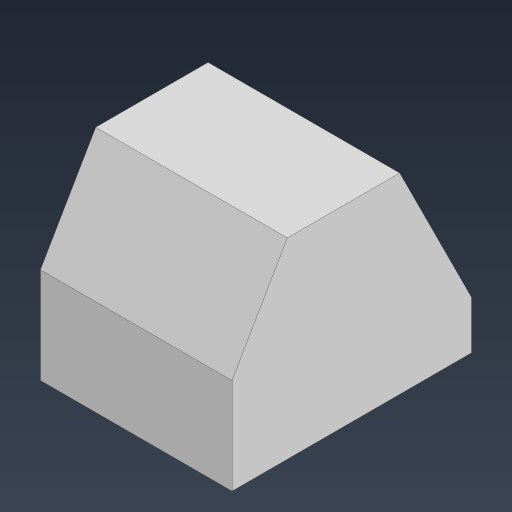
# Autodesk Inventor part: 3D Model
Saved by Autodesk Inventor 2024 (Build 280153000, 153)
## iProperties
Created: 2024-03-05
Part Number: 3D Model
Material: Genérico
Document SubType Name: Modeling
Designer: Administrator
Density: 1 g/cm^3
Appearance: Padrão
Author: Administrator
Autodesk Inventor part; units mm, degrees
ref_plane "YZ Plane" through (0, 0, 0) normal (1, 0, 0) x (0, 1, 0)
ref_plane "XZ Plane" through (0, 0, 0) normal (0, 1, 0) x (-1, 0, 0)
ref_plane "XY Plane" through (0, 0, 0) normal (0, 0, 1) x (1, 0, 0)
sketch "Esboço1" plane through (0, 0, 0) normal (0, 1, 0) x (-1, 0, 0)
  line L0 (20, -25) -> (-20, -25)
  line L1 (-20, -25) -> (-20, 25)
  line L2 (-20, 25) -> (20, 25)
  line L3 (20, 25) -> (20, -25)
  line L4 (20, -25) -> (-20, 25) construction
  line L5 (-20, -25) -> (20, 25) construction
  point P0 (0, 0)
  dimension "d0" = 40
  dimension "d1" = 50
  constraints: 12 end point, 2 midpoint, 2 parallel, 1 horizontal, 1 perpendicular
  measures "d0" distance of L1.end L2.end
  measures "d1" distance of L0.end L1.end
extrude "Extrusão1" add sketch "Esboço1" along normal blind 40
chamfer "Chanfro1" distance 20 angle 30 1 edges at (0, 40, 25) measured on face at (-6.6667, 13.3333, 25)
chamfer "Chanfro2" distance 15 distance2 30 1 edges at (0, 40, -25) measured on face at (6.6667, 40, 0.6353)
